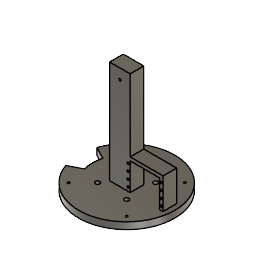
part - head base (Autodesk Fusion 360 design; units mm, degrees)
Autodesk Fusion 360 part; units mm, degrees
note: some values were not read from the file. Set by a fixed rule: which sketch regions a step uses.
sketch "Sketch1" plane through (0, 0, 0) normal (0, 1, 0) x (1, 0, 0)
  line L0 (15, -75) -> (-15, -75)
  line L1 (-15, -75) -> (-15, 75)
  line L2 (-15, 75) -> (15, 75)
  line L3 (15, 75) -> (15, -75)
  line L4 (15, -75) -> (-15, 75) construction
  line L5 (-15, -75) -> (15, 75) construction
  dimension "d1" = 150
  dimension "d2" = 30
  constraint horizontal L0
  constraint perpendicular L0 L1
  constraint parallel L0 L2
  constraint parallel L1 L3
  constraint coincident L4 origin
  constraint coincident L5 origin
  measures "d1" distance of L0.end L1.end
  measures "d2" distance of L0.start L0.end
extrude "Extrude1" add sketch "Sketch1" along normal blind 20 makes body 1
sketch "Sketch3" plane through (0, 0, -75) normal (0, 0, -1) x (1, 0, 0)
  line L0 (15, 0) -> (-15, 0)
  line L1 (-15, 0) -> (-15, -20)
  line L2 (-15, -20) -> (15, -20)
  line L3 (15, -20) -> (15, 0)
  line L4 (-15, -20) -> (15, 0)
  line L5 (15, -20) -> (-15, 0)
  circle A0 centre (0, -10) radius 70
  dimension "d5" = 140
  constraint coincident L1.end L2.start
  constraint coincident L0.start L3.end
  constraint coincident L2.end L3.start
  constraint coincident L0.end L1.start
  constraint midpoint L4 A0.centre
  measures "d5" diameter of A0
extrude "Extrude2" add sketch "Sketch3" along normal blind 10 separate body contours L0 L4 L5 | L3 L4 L5 | L1 L4 L5 | L2 L4 L5 | A0 makes body 2
sketch "Sketch4" plane through (0, 0, 0) normal (0, -1, 0) x (1, 0, 0)
  line L0 (-15, -75) -> (15, -75)
  line L1 (15, -75) -> (15, 75)
  line L2 (15, 75) -> (-15, 75)
  line L3 (-15, 75) -> (-15, -75)
  circle A0 centre (0, 60) radius 1.6
  dimension "d8" = 3.2
  dimension "d9" = 15
  dimension "d10" = 15
  measures "d8" diameter of A0
  measures "d9" distance of L2 A0.centre
  measures "d10" distance of L3 A0.centre
extrude "Extrude3" cut sketch "Sketch4" against normal blind 35 contours A0 bodies 1
sketch "Sketch5" plane through (15, 0, 0) normal (1, 0, 0) x (0, 1, 0)
  line L0 (0, 75) -> (0, -75)
  line L1 (0, -75) -> (20, -75)
  line L2 (20, -75) -> (20, 75)
  line L3 (20, 75) -> (0, 75)
  line L4 (19.9, -65.7145) -> (-0.1, -65.7145)
  line L5 (-0.1, -65.7145) -> (-0.1, -30)
  line L6 (-0.1, -30) -> (19.9, -30)
  line L7 (19.9, -30) -> (19.9, -65.7145)
  line L8 (19.9, -65.7145) -> (-0.1, -30) construction
  line L9 (-0.1, -65.7145) -> (19.9, -30) construction
  line L10 (-60, -75) -> (80, -75)
  line L11 (-60, -85) -> (80, -85)
  line L12 (-60, -75) -> (80, -75)
  line L13 (-0.1, -65.7145) -> (0, -75)
  line L14 (19.9, -65.7145) -> (20, -75)
  line L15 (-0.1, -35) -> (19.9, -35)
  point P0 (9.9, -47.8572)
  dimension "d13" = 20
  dimension "d14" = 45
  dimension "d15" = 5
  constraint horizontal L4
  constraint perpendicular L4 L5
  constraint parallel L4 L6
  constraint parallel L5 L7
  constraint coincident L8 P0
  constraint coincident L9 P0
  constraint coincident L0.end L1.start
  constraint coincident L1.end L2.start
  measures "d13" distance of L5.end L6.end
  measures "d14" distance of L6 L10
extrude "Extrude4" add sketch "Sketch5" along normal blind 48 contours L0 L6 L7 L15 bodies 1
sketch "Sketch6" plane through (0, 0, -35) normal (0, 0, -1) x (1, 0, 0)
  line L0 (15, 0) -> (15, -19.9)
  line L1 (63, -19.9) -> (63, 0)
  line L2 (63, 0) -> (15, 0)
  line L3 (58, 0) -> (63, 0)
  line L4 (63, -19.9) -> (58, -19.9)
  line L5 (63, -19.9) -> (63, 0)
  line L6 (15, -19.9) -> (63, -19.9)
  line L7 (15, -14.9) -> (58, -14.9)
  line L8 (58, -14.9) -> (58, 0)
  line L9 (58, -14.9) -> (58, -19.9)
  dimension "d18" = -5
  constraint coincident L1.end L2.start
  constraint perpendicular L1 L3
  constraint coincident L1.start L4.start
  constraint perpendicular L4 L8
  constraint perpendicular L4 L9
extrude "Extrude5" add sketch "Sketch6" along normal blind 40 contours L1 L2 L3 L4 L5 L6 L8 L9 bodies 1 2
sketch "Sketch7" plane through (0, 0, 0) normal (0, -1, 0) x (1, 0, 0)
  circle A0 centre (0, 60) radius 1.6
  line L0 (15, -75) -> (15, -35)
  line L1 (15, -35) -> (58, -35)
  line L2 (58, -35) -> (58, -75)
  line L3 (63, -75) -> (63, -30)
  line L4 (63, -30) -> (15, -30)
  line L5 (15, -30) -> (15, 75)
  line L6 (15, 75) -> (-15, 75)
  line L7 (-15, 75) -> (-15, -75)
  circle A1 centre (60.5, -69.5) radius 1.6
  line L8 (-70, -75) -> (70, -75)
  circle A2 centre (11.9, -69.5) radius 1.6
  circle A3 centre (60.5, -59.6) radius 1.6
  circle A4 centre (11.9, -59.6) radius 1.6
  circle A5 centre (11.9, -39.6) radius 1.6
  circle A6 centre (11.9, -49.5) radius 1.6
  circle A7 centre (60.5, -39.6) radius 1.6
  circle A8 centre (60.5, -49.5) radius 1.6
  line L9 (-15, -75) -> (15, -75)
  line L10 (58, -75) -> (63, -75)
  dimension "d21" = 3.2
  dimension "d22" = 5.5
  dimension "d23" = 2.5
  dimension "d26" = -48.6
  dimension "d27" = 9.9
  dimension "d30" = 0
  dimension "d31" = 20
  measures "d21" diameter of A1
  measures "d22" distance of A1.centre L8
  measures "d23" distance of L2 A1.centre
extrude "Extrude6" cut sketch "Sketch7" against normal blind 40 contours A1 | A2 | A3 | A4 | A5 | A6 | A7 | A8 bodies 1
sketch "Sketch9" plane through (0, 0, -75) normal (0, 0, 1) x (-1, 0, 0)
  line L0 (-63, 0) -> (-58, 0)
  line L1 (-58, 0) -> (-58, -19.9)
  line L2 (-58, -19.9) -> (-63, -19.9)
  line L3 (-63, -19.9) -> (-63, 0)
  circle A0 centre (0, -10) radius 70
  line L4 (15, 0) -> (15, -20)
  line L5 (15, -20) -> (-15, -20)
  line L6 (-15, -20) -> (-15, 0)
  line L7 (-15, 0) -> (15, 0)
  line L8 (-15, 0) -> (15, 0)
  circle A1 centre (21.2132, -31.2132) radius 3.25
  line L9 (0, -10) -> (21.2132, -31.2132)
  line L10 (-98.5462, -10) -> (98.5462, -10)
  circle A2 centre (21.2132, 11.2132) radius 3.25
  circle A3 centre (-21.2132, 11.2132) radius 3.25
  circle A4 centre (-21.2132, -31.2132) radius 3.25
  circle A5 centre (21.2132, -31.2132) radius 1.6
  circle A6 centre (21.2132, 11.2132) radius 1.6
  circle A7 centre (-21.2132, 11.2132) radius 1.6
  circle A8 centre (-21.2132, -31.2132) radius 1.6
  circle A9 centre (0, -10) radius 50
  circle A10 centre (-42.4264, 32.4264) radius 1.6
  line L11 (-42.4264, 32.4264) -> (0, -10)
  circle A11 centre (-42.4264, -52.4264) radius 1.6
  circle A12 centre (42.4264, -52.4264) radius 1.6
  circle A13 centre (42.4264, 32.4264) radius 1.6
  point P0 (21.2132, 11.2132)
  point P1 (-21.2132, 11.2132)
  point P2 (-21.2132, -31.2132)
  dimension "d48" = 6.5
  dimension "d53" = 30
  dimension "d54" = 45
  dimension "d56" = 360
  dimension "d57" = 3.2
  dimension "d58" = 100
  dimension "d63" = 3.2
  dimension "d64" = 60
  dimension "d65" = 45
  constraint coincident A0.centre L9.start
  constraint coincident A1.centre L9.end
  constraint midpoint A0.centre L10
  constraint horizontal L10
  constraint concentric A0 A9
  constraint coincident A10.centre L11.start
  measures "d48" diameter of A1
  measures "d53" distance of A0.centre A1.centre
  measures "d54" angle of L9 L10
  measures "d57" diameter of A5
  measures "d58" diameter of A9
  measures "d63" diameter of A10
  measures "d64" distance of A0.centre A10.centre
  measures "d65" angle of L10 L11
extrude "Extrude8" cut sketch "Sketch9" against normal blind 6.5 contours A3 A7 L11 | A3 A7 L11 | A1 | A2 | A4 bodies 1
extrude "Extrude9" cut 4 faces at (-21.6042, -11.576, -75) (20.8222, -11.576, -75) (20.8045, 30.7727, -75) (-21.4799, 30.7513, -75) along direction (0, 0, -1) blind 40 on bodies 1 bodies 1
extrude "Extrude11" cut sketch "Sketch9" against normal blind 30 contours A10 | A11 | A12 | A13 bodies 1
sketch "Sketch8" plane through (0, 0, -85) normal (0, 0, -1) x (1, 0, 0)
  circle A0 centre (21.2132, -31.2132) radius 1.6
  circle A1 centre (-21.2132, 11.2132) radius 1.6
  circle A2 centre (21.2132, 11.2132) radius 1.6
  circle A3 centre (-21.2132, -31.2132) radius 1.6
  circle A4 centre (0, -10) radius 70
  circle A5 centre (0, -10) radius 50
  circle A6 centre (0, -10) radius 11.5
  circle A7 centre (42.4264, -52.4264) radius 1.6
  circle A8 centre (42.4264, 32.4264) radius 1.6
  circle A9 centre (-42.4264, -52.4264) radius 1.6
  circle A10 centre (-42.4264, 32.4264) radius 1.6
  dimension "d59" = 100
  dimension "d60" = 23
  constraint concentric A4 A5
  constraint concentric A5 A6
  measures "d59" diameter of A5
  measures "d60" diameter of A6
extrude "Extrude7" cut sketch "Sketch8" against normal blind 3 contours A5 | A6 bodies 1
extrude "Extrude10" cut sketch "Sketch8" against normal blind 8.5 contours A6 bodies 1
sketch "Sketch10" plane through (0, 0, -75) normal (0, 0, 1) x (-1, 0, 0)
  circle A0 centre (-21.2132, -31.2132) radius 3.25
  circle A1 centre (-21.2132, 11.2132) radius 3.25
  circle A2 centre (21.2132, -31.2132) radius 3.25
  circle A3 centre (21.2132, 11.2132) radius 3.25
  line L0 (-63, 0) -> (-58, 0)
  line L1 (-58, 0) -> (-58, -19.9)
  line L2 (-58, -19.9) -> (-63, -19.9)
  line L3 (-63, -19.9) -> (-63, 0)
  circle A4 centre (0, -10) radius 70
  line L4 (15, 0) -> (15, -20)
  line L5 (15, -20) -> (-15, -20)
  line L6 (-15, -20) -> (-15, 0)
  line L7 (-15, 0) -> (15, 0)
  circle A5 centre (-42.4264, -52.4264) radius 1.6
  circle A6 centre (-42.4264, 32.4264) radius 1.6
  circle A7 centre (42.4264, -52.4264) radius 1.6
  circle A8 centre (42.4264, 32.4264) radius 1.6
  circle A9 centre (55, -10) radius 15
  circle A10 centre (42.4264, 32.4264) radius 1.6
  circle A11 centre (42.4264, -52.4264) radius 1.6
  circle A12 centre (-42.4264, 32.4264) radius 1.6
  circle A13 centre (-42.4264, -52.4264) radius 1.6
  circle A14 centre (0, -10) radius 70
  circle A15 centre (0, -10) radius 50
  line L8 (30.107, -14.1371) -> (66.2566, -32.5846)
  line L9 (30.107, -5.8629) -> (66.2566, 12.5846)
  point P0 (48.1818, -23.3609)
  point P1 (48.1818, 3.3609)
  dimension "d70" = 30
  dimension "d71" = 55
  constraint midpoint L8 P0
  constraint coincident A9 P0
  constraint coincident A15 P0
  constraint coincident A4 L8.end
  constraint tangent A9 L8
  constraint midpoint L9 P1
  constraint coincident A15 P1
  constraint coincident A9 P1
  constraint coincident A4 L9.end
  constraint tangent A9 L9
  measures "d70" diameter of A9
  measures "d71" distance of A4.centre A9.centre
extrude "Extrude12" cut sketch "Sketch10" against normal blind 100 contours A4 A9 A14 L9 | A9 A15 | A4 A9 A14 L8 picked at (55.7713, -5.744) bodies 1
equation "d14 = 20 mm + 20 mm + 5 mm"
equation "d61 = -3 mm - 5.5 mm"
